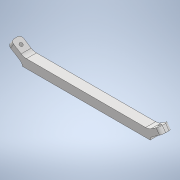
# Autodesk Inventor part: leg_switch_holder_1
Saved by Autodesk Inventor 2020 (Build 240168000, 168)
## iProperties
Created: 2019-08-05
Part Number: leg_switch_holder_1
Material: Generic
Document SubType Name: Modeling
Designer: psrob
Density: 1 g/cm^3
Appearance: Default
Author: psrob
Autodesk Inventor part; units mm, degrees
ref_plane "YZ Plane" through (0, 0, 0) normal (1, 0, 0) x (0, 1, 0)
ref_plane "XZ Plane" through (0, 0, 0) normal (0, 1, 0) x (-1, 0, 0)
ref_plane "XY Plane" through (0, 0, 0) normal (0, 0, 1) x (1, 0, 0)
sketch "Sketch1" plane through (0, 0, 0) normal (0, 0, 1) x (1, 0, 0)
  line L0 (96, 6.7) -> (90, 2.7) projected
  line L1 (10, 2.5) -> (2, 7.5) projected
  line L2 (0, 0) -> (100, 0) projected
  line L3 (96, 6.7) -> (96, 10.7) projected
  line L4 (2, 7.5) -> (3.855, 10.468)
  line L5 (96, 6.7) -> (94.0585, 9.6122)
  line L6 (94.0585, 9.6122) -> (87.4021, 5.1746)
  line L7 (3.855, 10.468) -> (12.3391, 5.1746)
  line L8 (87.4021, 5.1746) -> (12.3391, 5.1746)
  line L9 (90, 2.7) -> (88.3359, 1.5906)
  line L10 (88.3359, 1.5906) -> (88.3359, 0)
  line L11 (10, 2.5) -> (11.696, 1.44)
  line L12 (11.696, 1.44) -> (11.696, 0)
  line L13 (88.3359, 0) -> (11.696, 0)
  dimension "d0" = 3.5
  dimension "d1" = 3.5
  dimension "d2" = 8
  dimension "d3" = 10
  dimension "d4" = 2
  dimension "d5" = 2
  constraints: 20 end point, 3 collinear, 3 perpendicular, 2 point on line, 1 horizontal
  measures "d0" distance of L1.end L4.end
  measures "d1" distance of L0.start L5.end
  measures "d2" distance of L5.end L6.end
  measures "d3" distance of L4.end L7.end
  measures "d4" distance of L0.end L9.end
  measures "d5" distance of L1.start L11.end
ref_plane "Work Plane1" through (0, -6, -6) normal (0, 0, -1) x (0, 1, 0)
extrude "Extrusion1" add sketch "Sketch1" against normal up to surface (6 mm away)
sketch "Sketch2" plane through (87.4021, 5.1746, 0) normal (-0.5547002, 0.8320503, 0) x (0.8320503, 0.5547002, 0)
  circle A0 centre (4.3944, 3) radius 1 projected
  point P0 (-75.5933, 0)
extrude "Extrusion2" cut sketch "Sketch2" against normal blind 10
sketch "Sketch3" plane through (3.855, 10.468, 0) normal (0.529342, 0.8484086, 0) x (0.8484086, -0.529342, 0)
  ellipse E0 centre (4.7143, 3) end of major axis (4.7143, 2) minor radius 1 projected
  point P0 (2.2705, 0)
extrude "Extrusion3" cut sketch "Sketch3" against normal blind 10
fillet "Fillet1" radius 2 2 edges at (2.9275, 8.984, 0) (2.9275, 8.984, -6)
thicken "Thicken1" operation add thickness 1 both sides no extend neighbours yes toward (0.8479983, -0.5299989, 0) faces at (3.2367, 9.4787, -3.3333)
fillet "Fillet2" radius 2 2 edges at (95.0293, 8.1561, 0) (95.0293, 8.1561, -6)
thicken "Thicken2" operation add thickness 0.5 both sides no extend neighbours yes toward (-0.8320503, -0.5547002, 0) faces at (95.3528, 7.6707, -3.3333)
fillet "Fillet3" radius 6 2 edges at (87.4021, 5.1746, -3) (12.3391, 5.1746, -3)
fillet "Fillet4" radius 3 2 edges at (88.3359, 1.5906, -3) (11.696, 1.44, -3)
body "Solid1"
